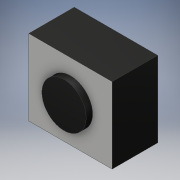
# Autodesk Inventor part: Button
Saved by Autodesk Inventor 2017 (Build 210142000, 142)
## iProperties
Created: 2016-08-05
Part Number: Button
Material: Generic
Document SubType Name: Modeling
Designer: ge937963
Density: 1 g/cm^3
Appearance: Glossy - Black
Author: ge937963
Autodesk Inventor part; units mm, degrees
ref_plane "YZ Plane" through (0, 0, 0) normal (1, 0, 0) x (0, 1, 0)
ref_plane "XZ Plane" through (0, 0, 0) normal (0, 1, 0) x (-1, 0, 0)
ref_plane "XY Plane" through (0, 0, 0) normal (0, 0, 1) x (1, 0, 0)
sketch "Sketch1" plane through (0, 0, 0) normal (0, 0, 1) x (1, 0, 0)
  line L0 (0, 5.9944) -> (6.604, 5.9944)
  line L1 (6.604, 5.9944) -> (6.604, 0)
  line L2 (6.604, 0) -> (0, 0)
  line L3 (0, 0) -> (0, 5.9944)
  dimension "d0" = 5.9944
  dimension "d1" = 6.604
  constraints: 8 end point, 2 parallel, 1 coincident, 1 horizontal, 1 perpendicular
  measures "d0" distance of L2.end L0.start
  measures "d1" distance of L0.start L0.end
extrude "Extrusion1" add sketch "Sketch1" along normal blind 3.6068
sketch "Sketch2" plane through (0, 0, 3.6068) normal (0, 0, 1) x (1, 0, 0)
  circle A0 centre (3.302, 2.9972) radius 1.7526
  line L0 (6.604, 5.9944) -> (0, 5.9944) projected
  line L1 (0, 5.9944) -> (0, 0) projected
  line L2 (0, 0) -> (6.604, 0) projected
  line L3 (6.604, 0) -> (6.604, 5.9944) projected
  point P0 (3.302, 5.9944)
  point P1 (6.604, 2.9972)
  dimension "d4" = 3.5052
  constraints: 2 midpoint, 1 centre point, 1 horizontal alignment, 1 vertical alignment
  measures "d4" diameter of A0
extrude "Extrusion2" add sketch "Sketch2" along normal blind 0.508 contours A0
body "Solid1"
